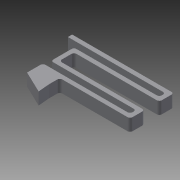
# Autodesk Inventor part: ValveRatcheKeep
Saved by Autodesk Inventor 2015 (Build 190159000, 159)
## iProperties
Created: 2016-01-09
Part Number: ValveRatcheKeep
Material: Generic
Document SubType Name: Modeling
Designer: HP USER
Density: 1 g/cm^3
Appearance: Default
Author: HP USER
Autodesk Inventor part; units mm, degrees
ref_plane "YZ Plane" through (0, 0, 0) normal (1, 0, 0) x (0, 1, 0)
ref_plane "XZ Plane" through (0, 0, 0) normal (0, 1, 0) x (-1, 0, 0)
ref_plane "XY Plane" through (0, 0, 0) normal (0, 0, 1) x (1, 0, 0)
sketch "Sketch1" plane through (0, 0, 0) normal (0, 0, 1) x (1, 0, 0)
  line L0 (-2.3872, 9.7109) -> (-0.4186, 9.7109) construction
  line L1 (1.082, 11.6795) -> (12.6128, 11.6795)
  line L2 (12.6128, 11.6795) -> (12.6128, 14.0795)
  line L3 (12.6128, 14.0795) -> (-1.3872, 14.0795)
  line L4 (-1.3872, 14.0795) -> (-1.3872, 16.4795)
  line L5 (-1.3872, 16.4795) -> (12.6128, 16.4795)
  line L6 (12.6128, 16.4795) -> (12.6128, 18.8795)
  line L7 (12.6128, 18.8795) -> (-2.0872, 18.8795)
  line L8 (-2.3872, 12.3795) -> (11.9128, 12.3795)
  line L9 (11.9128, 12.3795) -> (11.9128, 13.3795)
  line L10 (11.9128, 13.3795) -> (-2.0872, 13.3795)
  line L11 (-2.0872, 13.3795) -> (-2.0872, 17.1795)
  line L12 (-2.0872, 17.1795) -> (11.9128, 17.1795)
  line L13 (11.9128, 17.1795) -> (11.9128, 18.1795)
  line L14 (11.9128, 18.1795) -> (-2.0872, 18.1795)
  line L15 (-2.0872, 18.1795) -> (-2.0872, 18.8795)
  line L16 (1.2525, 8.0309) -> (-2.3872, 9.7739)
  line L17 (-2.3872, 9.7739) -> (-2.3872, 11.6795)
  line L18 (-2.3872, 11.6795) -> (-2.3872, 12.3795)
  line L19 (-1.9872, 17.0795) -> (12.0128, 17.0795)
  line L20 (12.0128, 17.0795) -> (12.0128, 18.2795)
  line L21 (12.0128, 18.2795) -> (-1.9872, 18.2795)
  line L22 (-1.9872, 18.2795) -> (-1.9872, 18.7795)
  line L23 (-1.9872, 18.7795) -> (12.5128, 18.7795)
  line L24 (12.5128, 18.7795) -> (12.5128, 16.5795)
  line L25 (12.5128, 16.5795) -> (-1.4872, 16.5795)
  line L26 (-1.4872, 16.5795) -> (-1.4872, 13.9795)
  line L27 (-1.4872, 13.9795) -> (12.5128, 13.9795)
  line L28 (12.5128, 13.9795) -> (12.5128, 11.7795)
  line L29 (1.082, 11.6795) -> (1.082, 9.913)
  line L30 (1.082, 9.913) -> (1.2525, 8.0309)
  dimension "d3" = 2.4
  dimension "d4" = 14
  dimension "d5" = 2.4
  dimension "d6" = 2.4
  dimension "d9" = 1
  dimension "d10" = 14
  dimension "d11" = 3.8
  dimension "d12" = 1
  constraints: 62 end point, 11 perpendicular, 4 point on line, 2 parallel, 1 horizontal, 1 vertical, 9 other
  measures "d3" distance of L1.end L2.end
  measures "d4" distance of L2.end L3.end
  measures "d5" distance of L3.end L4.end
  measures "d6" distance of L5.end L6.end
  measures "d9" distance of L8.end L9.end
  measures "d10" distance of L9.end L10.end
  measures "d11" distance of L10.end L11.end
  measures "d12" distance of L12.end L13.end
extrude "Extrusion1" add sketch "Sketch1" along normal blind 2
fillet "Fillet1" radius 0.4 14 edges at (-1.3872, 14.0795, 1) (-1.3872, 16.4795, 1) (-2.0872, 13.3795, 1) (-2.0872, 17.1795, 1) (11.9128, 13.3795, 1) (11.9128, 12.3795, 1) (12.6128, 11.6795, 1) (12.6128, 14.0795, 1) (12.6128, 16.4795, 1) (11.9128, 17.1795, 1) (11.9128, 18.1795, 1) (12.6128, 18.8795, 1) (1.082, 11.6795, 1) (-2.3872, 12.3795, 1)
sketch "Sketch2" plane through (-2.0872, 18.1795, 0) normal (-1, 0, 0) x (0, 0, 1)
  line L0 (0, 0) -> (0, 0.7) projected
  line L1 (0, 0) -> (2, 0) projected
  line L2 (2, 0.7) -> (2, 0) projected
  line L3 (0, 0.7) -> (2, 0.7) projected
  point P0 (0, -18.1795)
extrude "Extrusion2" add sketch "Sketch2" along normal blind 2
body "Solid1"
